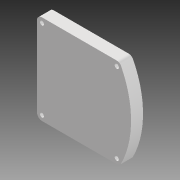
# Autodesk Inventor part: Bottom Case
Saved by Autodesk Inventor 2021 (Build 250183000, 183)
## iProperties
Created: 2022-08-24
Part Number: Bottom Case
Material: Generic
Document SubType Name: Modeling
Designer: Eli
Density: 1 g/cm^3
Appearance: Default
Author: Eli
Autodesk Inventor part; units mm, degrees
ref_plane "YZ Plane" through (0, 0, 0) normal (1, 0, 0) x (0, 1, 0)
ref_plane "XZ Plane" through (0, 0, 0) normal (0, 1, 0) x (-1, 0, 0)
ref_plane "XY Plane" through (0, 0, 0) normal (0, 0, 1) x (1, 0, 0)
sketch "Sketch1" plane through (0, 0, 0) normal (0, 0, 1) x (1, 0, 0)
  line L0 (-44.1613, -40) -> (-44.1613, 40) projected
  arc A0 (-39.1613, 45) -> (-44.1613, 40) centre (-39.1613, 40) ccw projected
  line L1 (-39.1613, 45) -> (35.8387, 45) projected
  arc A1 (39.8387, 43) -> (35.8387, 45) centre (35.8387, 40) ccw projected
  arc A2 (39.8387, -43) -> (39.8387, 43) centre (-44.1612, 0) ccw projected
  arc A3 (35.8387, -45) -> (39.8387, -43) centre (35.8387, -39.9999) ccw projected
  line L2 (35.8387, -45) -> (-39.1613, -45) projected
  arc A4 (-44.1613, -40) -> (-39.1613, -45) centre (-39.1613, -40) ccw projected
  circle A5 centre (-39.1613, -40) radius 2 projected
  circle A6 centre (-39.1613, 40) radius 2 projected
  circle A7 centre (35.8387, 40) radius 2.15 projected
  circle A8 centre (35.8387, -40) radius 2 projected
  arc A9 (37.5587, 41.29) -> (35.8387, 42.15) centre (35.8387, 40) ccw
  line L3 (35.8387, 42.15) -> (-39.1613, 42.15)
  arc A10 (-39.1613, 42.15) -> (-41.3113, 40) centre (-39.1613, 40) ccw
  line L4 (-41.3113, 40) -> (-41.3113, -40)
  arc A11 (-41.3113, -40) -> (-39.1613, -42.15) centre (-39.1613, -40) ccw
  line L5 (-39.1613, -42.15) -> (35.8387, -42.15)
  arc A12 (35.8387, -42.15) -> (37.5587, -41.29) centre (35.8387, -39.9999) ccw
  arc A13 (37.3698, -41.7362) -> (37.3698, 41.7362) centre (-44.1612, 0) ccw
  circle A14 centre (-39.1613, 40) radius 5
  circle A15 centre (35.8387, 40) radius 5
  circle A16 centre (35.8387, -40) radius 5
  circle A17 centre (-39.1613, -40) radius 5
  point P0 (0, 0)
  point P1 (39.8387, -43)
  point P2 (31.3246, 42.15)
  point P3 (39.7021, 36.826)
  point P4 (39.7021, -36.826)
  point P5 (31.3246, -42.15)
  point P6 (-34.6471, -42.15)
  point P7 (-41.3113, -35.4859)
  point P8 (-41.3113, 35.4859)
  point P9 (-34.6471, 42.15)
  constraints: 10 point on circle, 9 centre point, 6 end point, 4 coincident, 4 equal radius, 2 tangent, 6 other
extrude "Extrusion1" add sketch "Sketch1" along normal blind 8 contours A17 L4 A11 L5 A4 | L0 A14 L4 A17 | A0 A14 L3 A10 L4 | A17 L5 A16 L2 | A17 L5 A11 L4 | L1 A15 L3 A14 | L4 A10 L3 A14 | A16 A2 A3 | A1 A2 A15 A13 A7 L3 | L3 A7 A13 A15 | A16 A13 A15 A2
sketch "Sketch2" plane through (0, 0, 8) normal (0, 0, 1) x (1, 0, 0)
  arc A0 (-39.1613, 45) -> (-44.1613, 40) centre (-39.1613, 40) ccw projected
  line L0 (-44.1613, 40) -> (-44.1613, -40) projected
  arc A1 (-44.1613, -40) -> (-39.1613, -45) centre (-39.1613, -40) ccw projected
  line L1 (-39.1613, -45) -> (35.8387, -45) projected
  arc A2 (35.8387, -45) -> (39.8387, -43) centre (35.8387, -39.9999) ccw projected
  arc A3 (39.8387, -43) -> (39.8387, 43) centre (-44.1612, 0) ccw projected
  arc A4 (39.8387, 43) -> (35.8387, 45) centre (35.8387, 40) ccw projected
  line L2 (35.8387, 45) -> (-39.1613, 45) projected
  circle A5 centre (35.8387, 40) radius 2.15 projected
  circle A6 centre (35.8387, -40) radius 2 projected
  circle A7 centre (-39.1613, -40) radius 2 projected
  circle A8 centre (-39.1613, 40) radius 2 projected
  arc A9 (31.3246, 42.15) -> (39.7021, 36.826) centre (35.8387, 40) ccw projected
  arc A10 (39.7021, -36.826) -> (39.7021, 36.826) centre (-44.1612, 0) ccw projected
  arc A11 (39.7021, -36.826) -> (31.3246, -42.15) centre (35.8387, -40) ccw projected
  line L3 (31.3246, -42.15) -> (-34.6471, -42.15) projected
  arc A12 (-34.6471, -42.15) -> (-41.3113, -35.4859) centre (-39.1613, -40) ccw projected
  line L4 (-41.3113, -35.4859) -> (-41.3113, 35.4859) projected
  arc A13 (-41.3113, 35.4859) -> (-34.6471, 42.15) centre (-39.1613, 40) ccw projected
  line L5 (-34.6471, 42.15) -> (31.3246, 42.15) projected
  point P0 (0, 0)
extrude "Extrusion2" add sketch "Sketch2" along normal blind 4 contours L2 A4 A3 A2 L1 A1 L0 A0 | A9 A10 A11 L3 A12 L4 A13 L5
body "Solid1"
